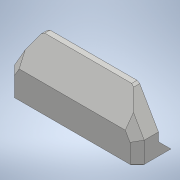
# Autodesk Inventor part: РучкаКрышки
Saved by Autodesk Inventor 2020 (Build 240168000, 168)
## iProperties
Created: 2021-05-21
Part Number: РучкаКрышки
Material: Типовые
Document SubType Name: Modeling
Designer: I_Love_U_Bogdan
Density: 1 g/cm^3
Appearance: По умолчанию
Author: I_Love_U_Bogdan
Autodesk Inventor part; units mm, degrees
ref_plane "YZ Plane" through (0, 0, 0) normal (1, 0, 0) x (0, 1, 0)
ref_plane "XZ Plane" through (0, 0, 0) normal (0, 1, 0) x (-1, 0, 0)
ref_plane "XY Plane" through (0, 0, 0) normal (0, 0, 1) x (1, 0, 0)
sketch "Эскиз1" plane through (0, 0, 0) normal (0, 0, 1) x (1, 0, 0)
  line L0 (54.2, 25) -> (95.8, 25) projected
  line L1 (54.2, 25) -> (54.2, 6.4142) projected
  line L2 (54.2, 6.4142) -> (55.9, 6.4142) projected
  line L3 (55.9, 5) -> (55.9, 6.4142) projected
  line L4 (94.1, 5) -> (55.9, 5) projected
  line L5 (94.1, 5) -> (94.1, 6.4142) projected
  line L6 (95.8, 6.4142) -> (94.1, 6.4142) projected
  line L7 (95.8, 25) -> (95.8, 6.4142) projected
  line L8 (78, 9.4569) -> (72, 9.4569) projected
  arc A0 (78, 6.4569) -> (78, 9.4569) centre (78, 7.9569) ccw projected
  line L9 (72, 6.4569) -> (78, 6.4569) projected
  arc A1 (72, 9.4569) -> (72, 6.4569) centre (72, 7.9569) ccw projected
  line L10 (52.2, 39.2872) -> (53.2, 35.5552) projected
  line L11 (52.2, 39.2872) -> (52.2, 10.774) projected
  line L12 (52.2, 10.774) -> (53.6142, 7.3598) projected
  line L13 (53.6142, 7.3598) -> (54.2, 6.774) projected
  line L14 (54.2, 6.774) -> (54.2, 8.5587) projected
  line L15 (54.2, 8.5587) -> (53.2, 10.9729) projected
  line L16 (53.2, 10.9729) -> (53.2, 35.5552) projected
  line L17 (97.8, 39.2872) -> (96.8, 35.5552) projected
  line L18 (96.8, 10.9729) -> (96.8, 35.5552) projected
  line L19 (95.8, 8.5587) -> (96.8, 10.9729) projected
  line L20 (95.8, 6.774) -> (95.8, 8.5587) projected
  line L21 (96.3858, 7.3598) -> (95.8, 6.774) projected
  line L22 (97.8, 10.774) -> (96.3858, 7.3598) projected
  line L23 (97.8, 39.2872) -> (97.8, 10.774) projected
  line L24 (53.6142, 7.3598) -> (54.2, 6.774) projected
  line L25 (10.2, 7.3598) -> (53.6142, 7.3598) projected
  line L26 (10.2, 1) -> (10.2, 7.3598) projected
  line L27 (10.2, 1) -> (139.8, 1) projected
  line L28 (139.8, 1) -> (139.8, 7.3598) projected
  line L29 (139.8, 7.3598) -> (96.3858, 7.3598) projected
  line L30 (96.3858, 7.3598) -> (95.8, 6.774) projected
  line L31 (95.8, 6.774) -> (95.8, 6.7) projected
  line L32 (95.8, 6.7) -> (94.1, 5) projected
  line L33 (94.1, 5) -> (55.9, 5) projected
  line L34 (54.2, 6.7) -> (55.9, 5) projected
  line L35 (54.2, 6.774) -> (54.2, 6.7) projected
  line L36 (93.2439, 7.3899) -> (87.9704, 16.5238)
  line L37 (62.7804, 16.9569) -> (87.2204, 16.9569)
  line L38 (56.7569, 7.3899) -> (62.0304, 16.5238)
  line L39 (87.2204, 16.9569) -> (87.9704, 16.5238)
  line L40 (62.7804, 16.9569) -> (62.0304, 16.5238)
  line L41 (72, 7.9569) -> (78, 7.9569)
  line L42 (56.7569, 7.3899) -> (56.7569, 1)
  line L43 (93.2439, 7.3899) -> (93.2439, 1)
  point P0 (0, 0)
  point P1 (75, 7.9569)
  dimension "d0" = 150
  dimension "d1" = 120
  dimension "d2" = 5.2735
  dimension "d3" = 9.567
  dimension "d4" = 23.517
  dimension "d5" = 31.5987
  dimension "d6" = 31.5987
  dimension "d7" = 9
  constraints: 16 end point, 4 perpendicular, 2 point on line, 1 horizontal, 1 midpoint
  measures "d0" angle of L39 L36
  measures "d1" angle of L37 L36
  measures "d2" distance from line of L36.start L39
  measures "d3" distance from line of L36.start L37
  measures "d4" distance from line of L36.start L40
  measures "d5" distance from line of L36.start L38
  measures "d6" distance from line of L38.start L36
  measures "d7" distance from line of L37 point (75, 7.957)
extrude "Выдавливание1" add sketch "Эскиз1" along normal blind 6 and the other way blind 4 contours L42 L38 L40 L37 L39 L36 L43 L4 | L4 L43 L27 L42 | A0 L9 A1 L8
sketch "Эскиз2" plane through (56.7569, 1, 6) normal (-1, 0, 0) x (0, 0, 1)
  line L0 (-6, 18.0421) -> (-6, 6.7284) projected
  line L1 (-10, 0) -> (-3.6402, 6.3598) projected
  line L2 (-6, 6.7284) -> (-6, 4)
  line L3 (-10, 15.5238) -> (0, 15.5238) projected
  line L4 (0, 15.9569) -> (0, 15.5238) projected
  line L5 (-10, 15.9569) -> (0, 15.9569) projected
  line L6 (-10, 15.5238) -> (-10, 15.9569) projected
  line L7 (-10, 6.3899) -> (0, 6.3899) projected
  line L8 (0, 15.5238) -> (0, 6.3899) projected
  line L9 (-10, 15.5238) -> (0, 15.5238) projected
  line L10 (-10, 6.3899) -> (-10, 15.5238) projected
  line L11 (-10, 0) -> (0, 0) projected
  line L12 (0, 6.3899) -> (0, 0) projected
  line L13 (-10, 6.3899) -> (0, 6.3899) projected
  line L14 (-10, 0) -> (-10, 6.3899) projected
  line L15 (0, 6.3899) -> (0, 15.5238) projected
  line L16 (0, 8.1626) -> (-4.5, 15.9569)
  line L17 (0, 15.9569) -> (-10, 15.9569) projected
  point P0 (-6, -1)
  point P1 (-6, 15.9569)
  dimension "d13" = 30
  dimension "d14" = 1.5
  constraints: 4 end point, 3 point on line, 1 vertical
  measures "d13" angle of L16 L8
  measures "d14" distance from line of L0 L16.end
extrude "Выдавливание2" cut sketch "Эскиз2" against normal through all contours L0 L3 L6 L5 | L0 L2 L7 L10 L3 | L5 L4 L3 L16 | L3 L8 L16 | L2 L1 L14 L7
chamfer "Фаска1" distance 2 angle 45 4 edges at (93.2439, 4.1949, 6) (56.7569, 4.1949, 6) (57.2686, 8.2762, 6) (92.7321, 8.2762, 6)
shell "Оболочка1" thickness 1 removed faces 1 at (80.4149, 1, -0.6667)
sketch "Эскиз3" plane through (57.7569, 4.5858, 1) normal (0, 0, 1) x (1, 0, 0)
  arc A0 (14.2431, 5.0711) -> (14.2431, 2.0711) centre (14.2431, 3.5711) ccw
  line L0 (20.2431, 5.0711) -> (14.2431, 5.0711)
  arc A1 (20.2431, 2.0711) -> (20.2431, 5.0711) centre (20.2431, 3.5711) ccw
  line L1 (14.2431, 2.0711) -> (20.2431, 2.0711)
  line L2 (35.487, 0.4142) -> (35.487, 2.8041) projected
  line L3 (-1, 0.4142) -> (35.487, 0.4142) projected
  line L4 (-1, 2.8041) -> (-1, 0.4142) projected
  line L5 (4.2735, 11.9381) -> (-1, 2.8041) projected
  line L6 (5.0235, 12.3711) -> (4.2735, 11.9381) projected
  line L7 (29.4635, 12.3711) -> (5.0235, 12.3711) projected
  line L8 (30.2135, 11.9381) -> (29.4635, 12.3711) projected
  line L9 (35.487, 2.8041) -> (30.2135, 11.9381) projected
  line L10 (20.2431, 4.8711) -> (14.2431, 4.8711) projected
  point P0 (-57.7569, -4.5858)
  point P1 (17.2435, 3.5711)
  dimension "d21" = 1.5
  dimension "d22" = 1.5
  dimension "d23" = 3.3538
  dimension "d24" = 6
  dimension "d25" = 0.2
  constraints: 4 end point, 4 point on circle, 3 tangent, 2 centre point, 1 equal radius, 1 parallel
  measures "d21" radius of A1
  measures "d22" distance from line of point (17.244, 3.571) L0
  measures "d23" distance of L0.start point (17.244, 3.571)
  measures "d24" distance of L0.end L0.start
  measures "d25" distance between parallel lines of L0 L10
extrude "Выдавливание3" cut sketch "Эскиз3" against normal blind 6 contours L0 A1 L1 A0
chamfer "Фаска2" distance 0.5 angle 45 5 edges at (75.0004, 1, 6) (56.7569, 1, 0) (57.7569, 1, 5) (93.2439, 1, 0) (92.2439, 1, 5)
